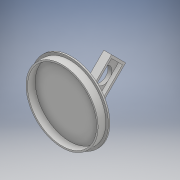
# Autodesk Inventor part: 第一關節
Saved by Autodesk Inventor 2017 (Build 210142000, 142)
## iProperties
Part Number: 第一關節
Material: 一般
Document SubType Name: Modeling
Designer: Brian
Density: 1 g/cm^3
Appearance: 預設
Author: Brian
Autodesk Inventor part; units mm, degrees
ref_plane "YZ Plane" through (0, 0, 0) normal (1, 0, 0) x (0, 1, 0)
ref_plane "XZ Plane" through (0, 0, 0) normal (0, 1, 0) x (-1, 0, 0)
ref_plane "XY Plane" through (0, 0, 0) normal (0, 0, 1) x (1, 0, 0)
sketch "草圖1" plane through (0, 0, 0) normal (0, 1, 0) x (-1, 0, 0)
  circle A0 centre (0, 0) radius 46.75
  circle A1 centre (0, 0) radius 44.75
  dimension "d0" = 93.5
  dimension "d1" = 2
  constraints: 2 centre point, 2 coincident
  measures "d0" diameter of A0
  measures "d1" radial gap between concentric circles of A0 A1
extrude "擠出1" add sketch "草圖1" along normal blind 10
sketch "草圖2" plane through (0, 10, 0) normal (0, 1, 0) x (1, 0, 0)
  circle A0 centre (0, 0) radius 50
  dimension "d4" = 100
  constraints: 1 centre point, 1 coincident
  measures "d4" diameter of A0
extrude "擠出2" add sketch "草圖2" along normal blind 2
sketch "草圖4" plane through (0, 0, 0) normal (1, 0, 0) x (0, 1, 0)
  line L0 (12, -50) -> (12, 50) projected
  line L1 (12, -25.0248) -> (30.0379, -25.0248)
  line L2 (30.0379, -25.0248) -> (30.0379, 11.7448)
  line L3 (30.0379, 11.7448) -> (12, 11.7448)
  line L4 (12, 11.7448) -> (12, -25.0248)
  line L5 (30.0379, -25.0248) -> (72.4644, 17.4017)
  line L6 (72.4644, 17.4017) -> (54.0796, 35.7864)
  line L7 (54.0796, 35.7864) -> (11.6532, -6.64)
  line L8 (11.6532, -6.64) -> (30.0379, -25.0248)
  point P0 (0, 0)
  dimension "d12" = 45
  dimension "d13" = 26
  dimension "d14" = 60
  constraints: 16 end point, 4 parallel, 2 perpendicular, 2 point on line, 1 horizontal
  measures "d12" angle of L2 L7
  measures "d13" distance of L5.end L6.end
  measures "d14" distance of L1.end L5.end
extrude "擠出4" add sketch "草圖4" along normal blind 5
fillet "圓角1" radius 10 1 edges at (2.5, 30.0379, 11.7448)
fillet "圓角2" radius 10 1 edges at (2.5, 30.0379, -25.0248)
sketch "草圖5" plane through (5, 0, 0) normal (1, 0, 0) x (0, 0, -1)
  line L0 (22.0958, 32.9669) -> (-17.4017, 72.4644) projected
  line L1 (-17.4017, 72.4644) -> (-35.7864, 54.0796) projected
  line L2 (-35.7864, 54.0796) -> (-14.6737, 32.9669) projected
  line L3 (20.7821, 30.0379) -> (-17.4017, 68.2217)
  line L4 (-17.4017, 68.2217) -> (-31.5438, 54.0796)
  line L5 (-31.5438, 54.0796) -> (-12.5524, 35.0882)
  line L6 (-31.5438, 54.0796) -> (-17.4017, 68.2217)
  line L7 (-17.4017, 68.2217) -> (20.7821, 30.0379)
  line L8 (20.7821, 30.0379) -> (6.64, 15.8958)
  line L9 (6.64, 15.8958) -> (-31.5438, 54.0796)
  arc A0 (25.0248, 25.8958) -> (22.0958, 32.9669) centre (15.0248, 25.8958) ccw projected
  line L10 (22.0958, 32.9669) -> (-17.4017, 72.4644) projected
  line L11 (-17.4017, 72.4644) -> (-35.7864, 54.0796) projected
  line L12 (-35.7864, 54.0796) -> (-14.6737, 32.9669) projected
  arc A1 (-11.7448, 25.8958) -> (-14.6737, 32.9669) centre (-21.7448, 25.8958) ccw projected
  line L13 (-11.7448, 25.8958) -> (-11.7448, 12) projected
  line L14 (25.0248, 12) -> (-11.7448, 12) projected
  line L15 (25.0248, 12) -> (25.0248, 25.8958) projected
  point P0 (0, 0)
  dimension "d19" = 20
  dimension "d20" = 54
  dimension "d21" = 54
  constraints: 14 end point, 3 equal length, 1 perpendicular, 2 other
  measures "d19" distance of L3.end L4.end
  measures "d20" distance of L3.start L3.end
  measures "d21" distance between parallel lines of L4 L8
extrude "擠出5" add sketch "草圖5" along normal blind 5
sketch "草圖6" plane through (0, 0, 0) normal (-1, 0, 0) x (0, 0, 1)
  circle A0 centre (12.4519, 49.1298) radius 10.5
  line L0 (12.4519, 49.1298) -> (26.594, 63.272)
  line L1 (17.4017, 72.4644) -> (35.7864, 54.0796) projected
  line L2 (-6.64, 15.8958) -> (-20.7821, 30.0379) projected
  point P0 (0, 0)
  dimension "d24" = 37
  dimension "d25" = 21
  constraints: 2 end point, 1 centre point, 1 midpoint, 1 perpendicular
  measures "d24" distance from line of L2 L0.start
  measures "d25" diameter of A0
extrude "擠出6" cut sketch "草圖6" against normal blind 5
